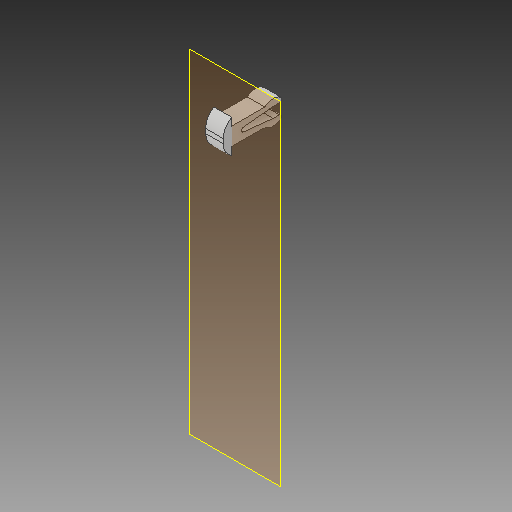
# Autodesk Inventor part: fastener
Saved by Autodesk Inventor 2017 (Build 210142000, 142)
## iProperties
Created: 2017-06-23
Part Number: fastener
Material: Generic
Document SubType Name: Modeling
Designer: erwin
Density: 1 g/cm^3
Appearance: Default
Author: erwin
Autodesk Inventor part; units mm, degrees
ref_plane "YZ Plane" through (0, 0, 0) normal (1, 0, 0) x (0, 1, 0)
ref_plane "XZ Plane" through (0, 0, 0) normal (0, 1, 0) x (-1, 0, 0)
ref_plane "XY Plane" through (0, 0, 0) normal (0, 0, 1) x (1, 0, 0)
ref_plane "Work Plane1" through (0, 0, 0) normal (0, 0, 1) x (1, 0, 0)
sketch "Sketch1" plane through (0, 0, 0) normal (0, 0, 1) x (1, 0, 0)
  circle A0 centre (-13, -7.5) radius 3 projected
  line L0 (-13, -7.5) -> (-10.8787, -9.6213) construction
  line L1 (-13, -7.5) -> (-10, -7.5) construction
  line L2 (-15.1213, -5.3787) -> (-10.8787, -5.3787)
  line L3 (-10.8787, -5.3787) -> (-10.8787, -9.6213)
  line L4 (-10.8787, -9.6213) -> (-15.1213, -9.6213)
  line L5 (-15.1213, -9.6213) -> (-15.1213, -5.3787)
  line L6 (-15.1213, -5.3787) -> (-10.8787, -9.6213) construction
  line L7 (-10.8787, -5.3787) -> (-15.1213, -9.6213) construction
  point P0 (0, 0)
  dimension "d0" = 45
  constraints: 16 end point, 2 horizontal, 2 midpoint, 2 parallel, 1 equal length, 1 perpendicular, 2 other
  measures "d0" angle of L0 L1
extrude "Extrusion1" add sketch "Sketch1" against normal blind 12 contours L3 L4 L5 L2
sketch "Sketch2" plane through (0, 0, 0) normal (0, 0, 1) x (1, 0, 0)
  circle A0 centre (-13, -7.5) radius 3 projected
  line L0 (-10.8787, -11.5) -> (-15.1213, -11.5)
  line L1 (-15.1213, -11.5) -> (-15.1213, -3.5)
  line L2 (-15.1213, -3.5) -> (-10.8787, -3.5)
  line L3 (-10.8787, -3.5) -> (-10.8787, -11.5)
  line L4 (-10.8787, -11.5) -> (-15.1213, -3.5) construction
  line L5 (-15.1213, -11.5) -> (-10.8787, -3.5) construction
  point P0 (0, 0)
  dimension "d3" = 8
  constraints: 12 end point, 2 midpoint, 2 parallel, 1 horizontal, 1 perpendicular
  measures "d3" distance of L0.end L1.end
extrude "Extrusion2" add sketch "Sketch2" along normal blind 2 contours L3 A0 L1 | A0 L1 L2 L3 | L3 L0 L1 A0
fillet "Fillet1" radius 4 2 edges at (-13, -3.5, 2) (-13, -11.5, 2)
sketch "Sketch3" plane through (-15.1213, -9.6213, -12) normal (-1, 0, 0) x (0, 0, 1)
  line L0 (4, 9.5928) -> (4, -5.4072) projected
  line L1 (12, 0) -> (0, 0) projected
  arc A0 (0, 0) -> (4, 0) centre (2, 2.2361) ccw
  line L2 (12, 4.2426) -> (0, 4.2426) projected
  arc A1 (4, 4.2426) -> (0, 4.2426) centre (2, 2.0066) ccw
  point P0 (12, 9.6213)
  dimension "d7" = 3
  dimension "d8" = 3
  constraints: 4 point on circle, 4 point on line, 2 centre point
  measures "d7" radius of A0
  measures "d8" radius of A1
extrude "Extrusion3" add sketch "Sketch3" against normal up to surface (4.2426 mm away)
sketch "Sketch4" plane through (-15.1213, -5.3787, 0) normal (-1, 0, 0) x (0, 0, 1)
  line L0 (-14, -3.3713) -> (-10, -3.3713)
  line L1 (-10, -3.3713) -> (-10, -0.8713)
  line L2 (-10, -0.8713) -> (-14, -0.8713)
  line L3 (-14, -0.8713) -> (-14, -3.3713)
  line L4 (-12, -4.2426) -> (-12, 0) projected
  line L5 (-14, -3.3713) -> (-10, -0.8713) construction
  line L6 (-10, -3.3713) -> (-14, -0.8713) construction
  line L7 (-10, -3.3713) -> (-2.7742, -2.6186)
  line L8 (2, -1.5854) -> (2, -2.6572) projected
  line L9 (-10, -0.8713) -> (-2.7742, -1.624)
  arc A0 (-2.7742, -2.6186) -> (-2.7742, -1.624) centre (-2.826, -2.1213) ccw
  point P0 (0, 5.3787)
  point P1 (-12, -2.1213)
  point P2 (2, -2.1213)
  dimension "d11" = 4
  dimension "d12" = 2.5
  dimension "d13" = 0.5
  constraints: 16 end point, 4 midpoint, 2 parallel, 2 point on circle, 2 point on line, 2 tangent, 1 centre point, 1 horizontal, 1 perpendicular
  measures "d11" distance of L2.end L1.end
  measures "d12" distance of L1.end L0.end
  measures "d13" radius of A0
extrude "Extrusion4" cut sketch "Sketch4" against normal up to next
fillet "Fillet2" radius 0.5 2 edges at (-13, -6.25, -12) (-13, -8.75, -12)
body "Solid1"
